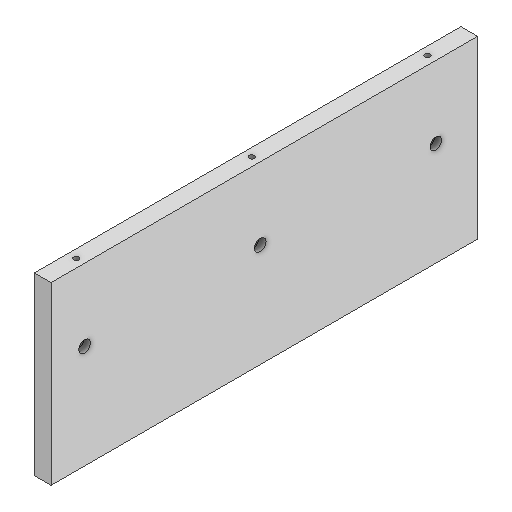
# Autodesk Inventor part: ER_Wand_1
Saved by Autodesk Inventor 2025.1 (Build 291241000, 241)
## iProperties
Created: 2025-06-25
Part Number: ER_Wand_1
Material: Generic
Document SubType Name: Modeling
Designer: Erik
Density: 1 g/cm^3
Appearance: Default
Author: Erik
Autodesk Inventor part; units mm, degrees
ref_plane "YZ Plane" through (0, 0, 0) normal (1, 0, 0) x (0, 1, 0)
ref_plane "XZ Plane" through (0, 0, 0) normal (0, 1, 0) x (-1, 0, 0)
ref_plane "XY Plane" through (0, 0, 0) normal (0, 0, 1) x (1, 0, 0)
sketch "Skizze1" plane through (0, 0, 0) normal (1, 0, 0) x (0, 1, 0)
  line L0 (-52.5, 127.5) -> (52.5, 127.5)
  line L1 (52.5, 127.5) -> (52.5, -127.5)
  line L2 (52.5, -127.5) -> (-52.5, -127.5)
  line L3 (-52.5, -127.5) -> (-52.5, 127.5)
  line L4 (-52.5, 127.5) -> (52.5, -127.5) construction
  line L5 (52.5, 127.5) -> (-52.5, -127.5) construction
  point P0 (0, 0)
  dimension "d0" = 105
  dimension "d1" = 255
  constraints: 12 end point, 2 midpoint, 2 parallel, 1 horizontal, 1 perpendicular
  measures "d0" distance of L1.end L2.end
  measures "d1" distance between parallel lines of L0 L2
extrude "Extrusion1" add sketch "Skizze1" along normal blind 10
sketch "Skizze2" plane through (10, 0, 0) normal (1, 0, 0) x (0, 0, -1)
  line L0 (-127.5, 52.5) -> (-127.5, -52.5) projected
  line L1 (127.5, -52.5) -> (127.5, 52.5) projected
  line L2 (127.5, 52.5) -> (-127.5, 52.5) projected
  point P0 (0, 0)
  point P1 (-107.5, 9.5)
  point P2 (-2.5, 9.5)
  point P3 (102.5, 9.5)
  dimension "d4" = 20
  dimension "d5" = 25
  dimension "d6" = 105
  dimension "d7" = 43
  dimension "d8" = 43
  dimension "d9" = 43
  measures "d4" distance from line of L0 point (-107.5, 9.5)
  measures "d5" distance from line of L1 point (102.5, 9.5)
  measures "d6" distance of point (-2.5, 9.5) point (102.5, 9.5)
  measures "d7" distance from line of L2 point (-107.5, 9.5)
  measures "d8" distance from line of point (-2.5, 9.5) L2
  measures "d9" distance from line of L2 point (102.5, 9.5)
hole "Bohrung1" at (10, 9.5, 107.5) at (10, 9.5, 2.5) at (10, 9.5, -102.5) direction (-1, 0, 0) diameter 3.242 end through all counterbore diameter 7 counterbore depth 4 thread size "M4x0.7" class "6H" standard "ISO Metric profile"
sketch "Skizze3" plane through (0, 52.5, 127.5) normal (0, 1, 0) x (1, 0, 0)
  line L0 (0, 0) -> (10, 0) projected
  line L1 (5, 0) -> (5, 250)
  line L2 (0, 255) -> (10, 255) projected
  point P0 (0, 127.5)
  point P1 (5, 20)
  point P2 (5, 125)
  point P3 (5, 230)
  point P4 (5, 255)
  dimension "d17" = 20
  dimension "d18" = 25
  dimension "d19" = 105
  constraints: 3 midpoint, 2 end point, 2 point on line, 1 vertical
  measures "d17" distance from line of L0 point (5, 20)
  measures "d18" distance of point (5, 230) point (5, 255)
  measures "d19" distance of point (5, 230) point (5, 125)
hole "Bohrung2" at (5, 52.5, 107.5) at (5, 52.5, 2.5) at (5, 52.5, -102.5) direction (0, -1, 0) diameter 3.242 depth 11.8 tip angle 118 thread size "M4x0.7" class "6H" standard "ISO Metric profile"
mirror "Spiegeln1" about plane through (0, 0, 0) normal (0, 1, 0) of "Bohrung2"
